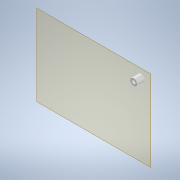
# Autodesk Inventor part: odroidstandoff
Saved by Autodesk Inventor 2020 (Build 240168000, 168)
## iProperties
Created: 2019-06-15
Part Number: odroidstandoff
Material: Generic
Document SubType Name: Modeling
Designer: amirt
Density: 1 g/cm^3
Appearance: Default
Author: amirt
Autodesk Inventor part; units mm, degrees
ref_plane "YZ Plane" through (0, 0, 0) normal (1, 0, 0) x (0, 1, 0)
ref_plane "XZ Plane" through (0, 0, 0) normal (0, 1, 0) x (-1, 0, 0)
ref_plane "XY Plane" through (0, 0, 0) normal (0, 0, 1) x (1, 0, 0)
ref_plane "Work Plane1" through (0, 0, 0) normal (0, 0, 1) x (1, 0, 0)
sketch "Sketch1" plane through (0, 0, 0) normal (0, 0, 1) x (1, 0, 0)
  circle A0 centre (76, 0) radius 1.4224 projected
  circle A1 centre (76, 0) radius 2.6924
  point P0 (0, 0)
  dimension "d2" = 1.27
  constraints: 1 centre point
  measures "d2" radial gap between concentric circles of A0 A1
extrude "Extrusion1" add sketch "Sketch1" along normal blind 6.096
body "Solid1"
